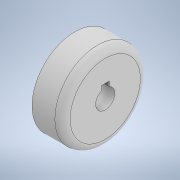
# Autodesk Inventor part: SpacerC
Saved by Autodesk Inventor 2021.2 (Build 252289000, 289)
## iProperties
Created: 2021-05-18
Part Number: SpacerC
Material: Generic
Document SubType Name: Modeling
Designer: Ryan
Density: 1 g/cm^3
Appearance: Default
Author: Ryan
Autodesk Inventor part; units mm, degrees
ref_plane "YZ Plane" through (0, 0, 0) normal (1, 0, 0) x (0, 1, 0)
ref_plane "XZ Plane" through (0, 0, 0) normal (0, 1, 0) x (-1, 0, 0)
ref_plane "XY Plane" through (0, 0, 0) normal (0, 0, 1) x (1, 0, 0)
sketch "Sketch1" plane through (0, 0, 0) normal (0, 0, 1) x (1, 0, 0)
  line L0 (0, 0) -> (0, 17.78)
  line L1 (0, 17.78) -> (9.525, 17.78)
  line L2 (12.7, 14.605) -> (12.7, 0)
  line L3 (12.7, 0) -> (0, 0)
  line L4 (0, 4) -> (12.7, 4)
  arc A0 (12.7, 14.605) -> (9.525, 17.78) centre (9.525, 14.605) ccw
  point P0 (12.7, 17.78)
  dimension "d0" = 17.78
  dimension "d1" = 12.7
  dimension "d2" = 4
  dimension "d3" = 3.175
  constraints: 10 end point, 4 perpendicular, 4 point on line, 2 point on circle, 2 tangent, 1 centre point, 1 vertical
  measures "d0" distance of L0.start L0.end
  measures "d1" distance of L0.end point (12.7, 17.78)
  measures "d2" distance between parallel lines of L3 L4
  measures "d3" radius of A0
revolve "Revolution1" add sketch "Sketch1" angle 360 about axis through (12.7, 0, 0) along (-1, 0, 0) contours L0 L1 A0 L2 L4
sketch "Sketch2" plane through (12.7, 0, 0) normal (1, 0, 0) x (0, 0, -1)
  line L0 (-1.5875, 5.5875) -> (1.5875, 5.5875)
  line L1 (1.5875, 5.5875) -> (1.5875, 2.4125)
  line L2 (1.5875, 2.4125) -> (-1.5875, 2.4125)
  line L3 (-1.5875, 2.4125) -> (-1.5875, 5.5875)
  circle A0 centre (0, 0) radius 4 projected
  line L4 (-1.5875, 5.5875) -> (1.5875, 2.4125) construction
  line L5 (1.5875, 5.5875) -> (-1.5875, 2.4125) construction
  point P0 (0, 4)
  dimension "d5" = 3.175
  dimension "d6" = 3.175
  constraints: 12 end point, 2 midpoint, 2 parallel, 1 horizontal, 1 perpendicular, 1 vertical alignment, 1 other
  measures "d5" distance of L1.end L2.end
  measures "d6" distance of L0.end L1.end
extrude "Extrusion1" cut sketch "Sketch2" against normal through all contours L0 L1 A0 L3 | A0 L1 L2 L3 picked at (0, 2.9417)
body "Solid1"
